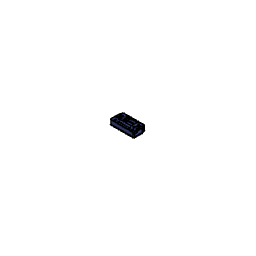
Remote (Autodesk Fusion 360 design; units mm, degrees)
Autodesk Fusion 360 part; units mm, degrees
(part 1 of 2)
sketch "Top" plane through (0, 0, 0) normal (0, 0, 1) x (1, 0, 0) in component "Case"
  line L0 (48, 28.17) -> (-50, 28.17) construction
  line L1 (-1, 28.17) -> (-1, -28.17) construction
  line L2 (-40, 26) -> (40, 26)
  circle A0 centre (45, -24.75) radius 3
  circle A1 centre (-47, -24.75) radius 1.3
  circle A2 centre (-47, -24.75) radius 3
  circle A3 centre (45, 24.75) radius 3
  line L3 (48, -28.17) -> (48, 28.17) construction
  circle A4 centre (-47, 24.75) radius 1.3
  line L4 (-50, -28.17) -> (48, -28.17) construction
  line L5 (40, 26) -> (40, -26)
  line L6 (40, -26) -> (-40, -26)
  circle A5 centre (45, -24.75) radius 1.3
  circle A6 centre (45, 24.75) radius 1.3
  line L7 (-40, -26) -> (-40, 26)
  line L8 (-50, 28.17) -> (-50, -28.17) construction
  circle A7 centre (-47, 24.75) radius 3
  line L9 (40, 0) -> (-40, 0) construction
  line L10 (-92, 15.5) -> (-92, -11.5) construction
  line L11 (-58, -11.5) -> (-92, 15.5) construction
  line L12 (-58, -11.5) -> (-58, 15.5) construction
  circle A8 centre (-75, 3) radius 11
  circle A9 centre (-62, -8) radius 2.5
  circle A10 centre (-88, -8) radius 2.5
  circle A11 centre (-88, 12) radius 2.5
  line L13 (-92, -11.5) -> (-58, -11.5) construction
  circle A12 centre (-88, 12) radius 1.25
  line L14 (-92, -11.5) -> (-58, 15.5) construction
  line L15 (-58, 2) -> (-92, 2) construction
  line L16 (-58, 15.5) -> (-92, 15.5) construction
  circle A13 centre (-62, 12) radius 1.25
  circle A14 centre (-88, -8) radius 1.25
  circle A15 centre (-62, -8) radius 1.25
  circle A16 centre (-62, 12) radius 2.5
  line L17 (-75, 15.5) -> (-75, -11.5) construction
  line L18 (1.75, 0) -> (22.5, 0)
  line L19 (0, 1.75) -> (0, 22.5)
  circle A17 centre (-45, -50) radius 3.625
  circle A18 centre (-45, -50) radius 9 construction
  line L20 (-75, 40) -> (-75, -70) construction
  circle A19 centre (-75, -50) radius 9 construction
  line L21 (-75, 10) -> (-75, -100) construction
  circle A20 centre (-75, -50) radius 3.625
  circle A21 centre (45, -50) radius 9 construction
  circle A22 centre (45, -50) radius 3.625
  circle A23 centre (75, -50) radius 9 construction
  circle A24 centre (75, -50) radius 3.625
  line L22 (-75, -50) -> (75, -50) construction
  circle A25 centre (-87, -23) radius 8
  circle A26 centre (-8, -50) radius 3.125
  circle A27 centre (87, -23) radius 8
  circle A28 centre (8, -50) radius 3.125
  line L23 (100, -65) -> (-100, -65)
  line L24 (-100, -65) -> (-100, 35)
  line L25 (-100, 35) -> (100, 35)
  line L26 (100, 35) -> (100, -65)
  line L27 (100, -65) -> (-100, 35) construction
  line L28 (-100, -65) -> (100, 35) construction
  circle A29 centre (62, -6) radius 2.5
  circle A30 centre (75, 5) radius 11
  line L29 (92, -9.5) -> (92, 17.5) construction
  circle A31 centre (88, 14) radius 1.25
  circle A32 centre (88, 14) radius 2.5
  line L30 (58, 17.5) -> (58, -9.5) construction
  circle A33 centre (88, -6) radius 2.5
  line L31 (58, -9.5) -> (92, -9.5) construction
  circle A34 centre (88, -6) radius 1.25
  line L32 (58, -9.5) -> (92, 17.5) construction
  circle A35 centre (62, 14) radius 2.5
  line L33 (92, 17.5) -> (58, 17.5) construction
  line L34 (92, 4) -> (58, 4) construction
  circle A36 centre (62, 14) radius 1.25
  line L35 (75, 17.5) -> (75, -9.5) construction
  circle A37 centre (62, -6) radius 1.25
  line L36 (92, -9.5) -> (58, 17.5) construction
  circle A38 centre (-63, -23) radius 8
  circle A39 centre (63, -23) radius 8
  circle A40 centre (-23, -50) radius 3.125
  circle A41 centre (23, -50) radius 3.125
  circle A42 centre (-55, 25) radius 3.125
  circle A43 centre (55, 25) radius 3.125
  line L37 (-43.5, -42.95) -> (-46.5, -42.95)
  line L38 (-46.5, -42.95) -> (-46.5, -41.45)
  line L39 (-46.5, -41.45) -> (-43.5, -41.45)
  line L40 (-43.5, -41.45) -> (-43.5, -42.95)
  line L41 (-43.5, -42.95) -> (-46.5, -41.45) construction
  line L42 (-46.5, -42.95) -> (-43.5, -41.45) construction
  line L43 (-36.45, -51.5) -> (-37.95, -51.5)
  line L44 (-37.95, -51.5) -> (-37.95, -48.5)
  line L45 (-37.95, -48.5) -> (-36.45, -48.5)
  line L46 (-36.45, -48.5) -> (-36.45, -51.5)
  line L47 (-36.45, -51.5) -> (-37.95, -48.5) construction
  line L48 (-37.95, -51.5) -> (-36.45, -48.5) construction
  line L49 (-43.5, -58.55) -> (-43.5, -57.05)
  line L50 (-46.5, -58.55) -> (-43.5, -58.55)
  line L51 (-46.5, -57.05) -> (-46.5, -58.55)
  line L52 (-43.5, -57.05) -> (-46.5, -57.05)
  line L53 (-73.75, -44.25) -> (-76.25, -44.25)
  line L54 (-76.25, -44.25) -> (-76.25, -42.75)
  line L55 (-76.25, -42.75) -> (-73.75, -42.75)
  line L56 (-73.75, -42.75) -> (-73.75, -44.25)
  line L57 (-73.75, -44.25) -> (-76.25, -42.75) construction
  line L58 (-76.25, -44.25) -> (-73.75, -42.75) construction
  line L59 (-45, -59) -> (-45, -41) construction
  line L60 (-52.05, -48.5) -> (-53.55, -48.5)
  line L61 (-52.05, -51.5) -> (-52.05, -48.5)
  line L62 (-53.55, -48.5) -> (-53.55, -51.5)
  line L63 (-53.55, -51.5) -> (-52.05, -51.5)
  line L64 (0, 1.75) -> (0, 22.5) construction
  line L65 (76.25, -42.75) -> (73.75, -42.75)
  line L66 (76.25, -44.25) -> (76.25, -42.75)
  line L67 (73.75, -44.25) -> (76.25, -44.25)
  line L68 (73.75, -42.75) -> (73.75, -44.25)
  line L69 (46.5, -41.45) -> (43.5, -41.45)
  line L70 (46.5, -42.95) -> (46.5, -41.45)
  line L71 (43.5, -42.95) -> (46.5, -42.95)
  line L72 (43.5, -41.45) -> (43.5, -42.95)
  line L73 (37.95, -51.5) -> (37.95, -48.5)
  line L74 (36.45, -48.5) -> (36.45, -51.5)
  line L75 (37.95, -48.5) -> (36.45, -48.5)
  line L76 (36.45, -51.5) -> (37.95, -51.5)
  line L77 (52.05, -51.5) -> (52.05, -48.5)
  line L78 (52.05, -48.5) -> (53.55, -48.5)
  line L79 (53.55, -48.5) -> (53.55, -51.5)
  line L80 (53.55, -51.5) -> (52.05, -51.5)
  line L81 (43.5, -57.05) -> (46.5, -57.05)
  line L82 (46.5, -57.05) -> (46.5, -58.55)
  line L83 (46.5, -58.55) -> (43.5, -58.55)
  line L84 (43.5, -58.55) -> (43.5, -57.05)
  line L85 (-87, -23) -> (-63, -23) construction
  line L86 (82, -43) -> (68, -43)
  line L87 (68, -43) -> (68, -57)
  line L88 (68, -57) -> (82, -57)
  line L89 (82, -57) -> (82, -43)
  line L90 (82, -43) -> (68, -57) construction
  line L91 (68, -43) -> (82, -57) construction
  line L92 (-68, -57) -> (-82, -57)
  line L93 (-68, -43) -> (-68, -57)
  line L94 (-82, -57) -> (-82, -43)
  line L95 (-82, -43) -> (-68, -43)
  point P0 (-75, 2)
  point P1 (-75, 2)
  point P2 (0, -15)
  point P3 (75, 4)
  point P4 (75, 4)
  point P5 (74.877, 10)
  point P6 (-45, -42.2)
  point P7 (-37.2, -50)
  point P8 (-75, -43.5)
  point P9 (75, -50)
  dimension "d1592" = 80
  dimension "d1593" = 52
  dimension "d1594" = 98
  dimension "d1595" = 56.34
  dimension "d1596" = 2.6
  dimension "d1597" = 3.42
  dimension "d1598" = 3
  dimension "d1607" = 6
  dimension "d1608" = 34
  dimension "d1609" = 27
  dimension "d1610" = 5
  dimension "d1611" = 2.5
  dimension "d1612" = 10
  dimension "d1613" = 13
  dimension "d1614" = 22
  dimension "d1615" = 1
  dimension "d1616" = 28.17
  dimension "d1617" = 50
  dimension "d1618" = 40
  dimension "d1619" = 35
  dimension "d1629" = 7.25
  dimension "d1630" = 18
  dimension "d1632" = 7.25
  dimension "d1633" = 18
  dimension "d1634" = 16
  dimension "d1635" = 6.25
  dimension "d1638" = 30
  dimension "d1641" = 200
  dimension "d1642" = 100
  dimension "d1650" = 32
  dimension "d1651" = 15
  dimension "d1652" = 35
  dimension "d1653" = 34
  dimension "d1654" = 27
  dimension "d1655" = 5
  dimension "d1656" = 2.5
  dimension "d1657" = 10
  dimension "d1658" = 13
  dimension "d1659" = 22
  dimension "d1660" = 1
  dimension "d1661" = 35
  dimension "d1817" = 12
  dimension "d1819" = 58
  dimension "d1820" = 25
  dimension "d1821" = 6.25
  dimension "d1822" = 22
  dimension "d1823" = 15
  dimension "d1824" = 6.25
  dimension "d1825" = 10
  dimension "d1826" = 45
  dimension "d1853" = 3
  dimension "d1854" = 1.5
  dimension "d1855" = 7.8
  dimension "d1856" = 1.5
  dimension "d1857" = 3
  dimension "d1858" = 7.8
  dimension "d1859" = 2.5
  dimension "d1860" = 1.5
  dimension "d1861" = 6.5
  dimension "d1864" = 14
  dimension "d1865" = 14
  constraint horizontal L2
  constraint vertical L5
  constraint horizontal L6
  constraint vertical L7
  constraint midpoint L9.start L5
  constraint midpoint L9.end L7
  constraint horizontal L0
  constraint perpendicular L0 L8
  constraint parallel L0 L4
  constraint parallel L3 L8
  constraint symmetric A5 A6 L9
  constraint concentric A0 A5
  constraint symmetric A0 A3 L9
  constraint midpoint L1.start L0
  constraint midpoint L1.end L4
  constraint symmetric L1 A1 A5
  constraint symmetric L1 A4 A6
  constraint symmetric L1 A0 A2
  constraint symmetric L1 A3 A7
  constraint perpendicular L12 L13
  constraint parallel L13 L16
  constraint parallel L10 L12
  constraint concentric A9 A15
  constraint symmetric A9 A10 L17
  constraint symmetric A14 A15 L17
  constraint symmetric A9 L15 A16
  constraint symmetric L15 A13 A15
  constraint symmetric A10 A11 L15
  constraint symmetric A12 L15 A14
  constraint coincident A8.centre L17
  constraint coincident P1 L11
  constraint coincident P1 L14
  constraint coincident P1 L17
  constraint coincident L17.end L13
  constraint coincident L17.start L16
  constraint coincident L15.end L10
  constraint coincident L15.start L12
  constraint coincident P1 L15
  constraint perpendicular L10 L15
  constraint collinear L9 L18
  constraint concentric A17 A18
  constraint vertical L20
  constraint concentric A19 A20
  constraint vertical L21
  constraint symmetric L19 A17 A22
  constraint symmetric L19 A18 A21
  constraint symmetric L19 A19 A23
  constraint symmetric L19 A20 A24
  constraint coincident A19.centre A20.centre
  constraint coincident P9 A23.centre
  constraint coincident L22 A26.centre
  constraint coincident A17.centre L22
  constraint coincident L21 A19.centre
  constraint symmetric L19 A25 A27
  constraint symmetric L19 A26 A28
  constraint horizontal L23
  constraint perpendicular L23 L24
  constraint parallel L23 L25
  constraint parallel L24 L26
  constraint coincident L27 P2
  constraint coincident L28 P2
  constraint coincident L19 P2
  constraint parallel L10 L17
  constraint parallel L13 L18
  constraint perpendicular L29 L31
  constraint parallel L31 L33
  constraint parallel L29 L30
  constraint concentric A33 A34
  constraint symmetric A29 A33 L35
  constraint symmetric A34 L35 A37
  constraint symmetric A32 A33 L34
  constraint symmetric A31 A34 L34
  constraint symmetric A29 A35 L34
  constraint symmetric L34 A36 A37
  constraint coincident A30.centre L35
  constraint coincident P4 L36
  constraint coincident P4 L32
  constraint coincident P4 L35
  constraint coincident L35.end L31
  constraint coincident L35.start L33
  constraint coincident L34.end L30
  constraint coincident L34.start L29
  constraint coincident P4 L34
  constraint perpendicular L30 L34
  constraint parallel L30 L35
  constraint collinear L20 L21
  constraint symmetric L20 A25 A38
  constraint symmetric L19 A38 A39
  constraint coincident L22 A40.centre
  constraint symmetric L19 A40 A41
  constraint symmetric L19 A42 A43
  constraint horizontal L37
  constraint perpendicular L37 L38
  constraint parallel L37 L39
  constraint parallel L38 L40
  constraint coincident L41 P6
  constraint coincident L42 P6
  constraint horizontal L43
  constraint perpendicular L43 L44
  constraint parallel L43 L45
  constraint parallel L44 L46
  constraint coincident L47 P7
  constraint coincident L48 P7
  constraint coincident L22 P7
  constraint symmetric L22 L37.start L49.end
  constraint symmetric L22 L37.end L51.start
  constraint symmetric L22 L38.end L50.start
  constraint symmetric L22 L39.end L49.start
  constraint horizontal L53
  constraint perpendicular L53 L54
  constraint parallel L53 L55
  constraint parallel L54 L56
  constraint coincident L57 P8
  constraint coincident L58 P8
  constraint coincident L20 P8
  constraint coincident L21 P8
  constraint coincident A18 L59.start
  constraint coincident A18 L59.end
  constraint perpendicular L39 L59
  constraint symmetric L43.start L59 L62.end
  constraint symmetric L43.end L59 L61.start
  constraint symmetric L44.end L59 L60.start
  constraint symmetric L45.end L59 L60.end
  constraint symmetric L37.start L64 L71.start
  constraint symmetric L37.end L64 L70.start
  constraint symmetric L38.end L64 L69.start
  constraint symmetric L39.end L64 L69.end
  constraint symmetric L43.start L64 L74.end
  constraint symmetric L43.end L64 L73.start
  constraint symmetric L44.end L64 L73.end
  constraint symmetric L45.end L64 L74.start
  constraint symmetric L49.start L64 L83.end
  constraint symmetric L49.end L64 L81.start
  constraint symmetric L50.start L64 L82.end
  constraint symmetric L51.start L64 L81.end
  constraint symmetric L53.start L64 L67.start
  constraint symmetric L53.end L64 L66.start
  constraint symmetric L54.end L64 L65.start
  constraint symmetric L55.end L64 L65.end
  constraint symmetric L60.start L64 L77.end
  constraint symmetric L60.end L64 L78.end
  constraint symmetric L61.start L64 L77.start
  constraint symmetric L62.end L64 L79.end
  constraint coincident A25.centre L85.start
  constraint coincident A38.centre L85.end
  constraint horizontal L86
  constraint perpendicular L86 L87
  constraint parallel L86 L88
  constraint parallel L87 L89
  constraint coincident L90 P9
  constraint coincident L91 P9
  constraint symmetric L19 L86.start L94.end
  constraint symmetric L19 L86.end L93.start
  constraint symmetric L19 L87.end L92.start
  constraint symmetric L19 L88.end L92.end
  measures "d1592" distance of L2.start L2.end
  measures "d1593" distance of L2.start L6.end
  measures "d1594" distance of L3.start L4.start
  measures "d1595" distance of L0.end L4.start
  measures "d1596" diameter of A5
  measures "d1597" distance of A0.centre L4
  measures "d1598" distance of A0.centre L3
  measures "d1607" diameter of A0
  measures "d1608" distance of L12.end L10.start
  measures "d1609" distance of L12.end L11.start
  measures "d1610" diameter of A9
  measures "d1611" diameter of A15
  measures "d1612" distance of A9.centre L15
  measures "d1613" distance of A9.centre L17
  measures "d1614" diameter of A8
  measures "d1615" distance of A8.centre L15
  measures "d1616" distance of L0 L9
  measures "d1617" distance of L8 L19
  measures "d1618" distance of L7 L19
  measures "d1619" distance of L7 A8.centre
  measures "d1629" diameter of A17
  measures "d1630" diameter of A18
  measures "d1632" diameter of A20
  measures "d1633" diameter of A19
  measures "d1634" diameter of A25
  measures "d1635" diameter of A26
  measures "d1638" distance of A17.centre A19.centre
  measures "d1641" distance of L24.end L25.end
  measures "d1642" distance of L23.end L24.end
  measures "d1650" distance of A8.centre L25
  measures "d1651" distance of L22 L23
  measures "d1652" distance of L9 L25
  measures "d1653" distance of L30.start L29.end
  measures "d1654" distance of L29.start L29.end
  measures "d1655" diameter of A33
  measures "d1656" diameter of A34
  measures "d1657" distance of A33.centre L34
  measures "d1658" distance of A33.centre L35
  measures "d1659" diameter of A30
  measures "d1660" distance of A30.centre L34
  measures "d1661" distance of L5 A30.centre
  measures "d1817" distance of L20 A25.centre
  measures "d1819" distance of A25.centre L25
  measures "d1820" distance of L20 L24
  measures "d1821" diameter of A40
  measures "d1822" distance of A17.centre A40.centre
  measures "d1823" distance of A26.centre A40.centre
  measures "d1824" diameter of A42
  measures "d1825" distance of L25 A42.centre
  measures "d1826" distance of L24 A42.centre
  measures "d1853" distance of L38.end L39.end
  measures "d1854" distance of L37.end L38.end
  measures "d1855" distance of A17.centre P6
  measures "d1856" distance of L44.end L45.end
  measures "d1857" distance of L43.end L44.end
  measures "d1858" distance of A17.centre P7
  measures "d1859" distance of L54.end L55.end
  measures "d1860" distance of L53.end L54.end
  measures "d1861" distance of A19.centre P8
  measures "d1864" distance of L87.end L88.end
  measures "d1865" distance of L86.end L87.end
extrude "Extrude1" add sketch "Top" against normal blind 38 contours L2 L5 L6 L7 | A0 | A1 | A2 | A3 | A4 | A5 | A6 | A7 | A8 | A9 | A10 | A11 | A12 | A13 | A14 | A15 | A16 | A17 | A20 | A22 | A24 | A25 | A26 | A27 | A28 | L23 L24 L25 L26 | A29 | A30 | A31 | A32 | A33 | A34 | A35 | A36 | A37 | A38 | A39 | A40 | A41 | A42 | A43 | L37 L38 L39 L40 | L43 L44 L45 L46 | L49 L50 L51 L52 | L53 L54 L56 L92 L93 L94 L95 | L53 L54 L56 L95 | L54 L55 L56 L95 | L60 L61 L62 L63 | L65 L66 L68 L86 | L66 L67 L68 L86 L87 L88 L89 | L66 L67 L68 L86 | L69 L70 L71 L72 | L73 L74 L75 L76 | L77 L78 L79 L80 | L81 L82 L83 L84 makes body 1 in component "Case"
sketch "Front" plane through (0, -65, 0) normal (0, -1, 0) x (1, 0, 0) in component "Case"
  line L0 (100, 0) -> (-100, 0)
  line L1 (-100, 0) -> (-100, -38)
  line L2 (-100, -38) -> (100, -38)
  line L3 (100, -38) -> (100, 0)
  circle A0 centre (97.5, -10) radius 2.5
  line L4 (100, 0) -> (100, -38) construction
  line L5 (100, 0) -> (0, 0) construction
  circle A1 centre (97.5, -10) radius 3.7
  line L6 (93.8001, -10.0324) -> (93.8001, 0)
  dimension "d1842" = 5
  dimension "d1843" = 2.5
  dimension "d1844" = 10
  dimension "d1845" = 7.4
  constraint coincident L0.start L3.end
  constraint coincident L2.end L3.start
  constraint coincident L5.end origin
  constraint concentric A0 A1
  constraint vertical L6
  constraint coincident A1 L6.start
  constraint coincident L5 L6.end
  measures "d1842" diameter of A0
  measures "d1843" distance of A0.centre L4
  measures "d1844" distance of A0.centre L5
  measures "d1845" diameter of A1
chamfer "Chamfer2" distance 10 distance2 30 1 edges at (100, 35, -19) measured on face at (-33.3333, 35, -12.6667) on bodies 1 in component "Case"
chamfer "Chamfer3" distance 30 distance2 10 1 edges at (-100, 35, -19) measured on face at (-100, -31.6667, -12.6667) on bodies 1 in component "Case"
fillet "Fillet4" radius 5 6 edges at (100, -65, -19) (-100, -65, -19) (90, 35, -19) (100, 5, -19) (-90, 35, -19) (-100, 5, -19) on bodies 1 in component "Case"
shell "Shell1" thickness 2.7 outward yes removed faces 1 at (31.6667, -18.8743, -38) on bodies 1 in component "Case"
extrude "Extrude2" cut sketch "Top" along normal blind 10 contours L2 L5 L6 L7 | A8 | A17 | A20 | A22 | A24 | A25 | A26 | A27 | A28 | A30 | A38 | A39 | A40 | A41 | A42 | A43 bodies 1 in component "Case"
extrude "Extrude4" add sketch "Top" against normal blind 4 contours A0 | A2 | A3 | A7 bodies 1 in component "Case"
extrude "Extrude5" add sketch "Top" against normal blind 17 contours A9 | A10 | A11 | A16 | A29 | A32 | A33 | A35 bodies 1 in component "Case"
extrude "Extrude15" cut sketch "Top" along normal blind 2.1 contours L37 L38 L39 L40 | L43 L44 L45 L46 | L49 L50 L51 L52 | L53 L54 L56 L95 | L54 L55 L56 L95 | L60 L61 L62 L63 | L65 L66 L68 L86 | L66 L67 L68 L86 | L69 L70 L71 L72 | L73 L74 L75 L76 | L77 L78 L79 L80 | L81 L82 L83 L84 bodies 1 in component "Case"
extrude "Extrude16" add sketch "Top" against normal blind 1.8 contours L53 L54 L56 L92 L93 L94 L95 | L66 L67 L68 L86 L87 L88 L89 bodies 1 in component "Case"
sketch "Left" plane through (-100, 0, 0) normal (1, 0, 0) x (0, 1, 0) in component "Case"
  line L0 (4.1886, 0) -> (-60, 0)
  line L1 (-60, -38) -> (4.1886, -38)
  line L2 (-60, 0) -> (4.1886, 0) construction
  line L3 (4.1886, 0) -> (4.1886, -38) construction
  line L4 (4.1886, -38) -> (-60, -38) construction
  line L5 (-60, -38) -> (-60, 0) construction
  line L6 (-37.9057, -38) -> (-17.9057, -38)
  line L7 (-17.9057, -38) -> (-17.9057, -32.6)
  line L8 (-17.9057, -32.6) -> (-37.9057, -32.6)
  line L9 (-37.9057, -32.6) -> (-37.9057, -38)
  line L10 (-60, 0) -> (-60, -38)
  line L11 (4.1886, -38) -> (4.1886, 0)
  point P0 (-27.9057, -38)
  point P1 (-27.9057, -38)
  dimension "d1712" = 20
  dimension "d1713" = 5.4
  constraint horizontal L2
  constraint vertical L3
  constraint horizontal L4
  constraint vertical L5
  constraint coincident L1.end L3.end
  constraint coincident L0.end L2.start
  constraint horizontal L6
  constraint vertical L7
  constraint horizontal L8
  constraint vertical L9
  constraint coincident L4 L6.start
  constraint midpoint L6 P1
  constraint midpoint L4 P1
  constraint coincident P1 P0
  measures "d1712" distance of L6.start L6.end
  measures "d1713" distance of L6.start L8.end
sketch "Back" plane through (0, 35, 0) normal (0, -1, 0) x (1, 0, 0) in component "Case"
  line L0 (86.3962, 0) -> (-86.3962, 0)
  line L1 (-86.3962, -38) -> (86.3962, -38)
  line L2 (-86.3962, 0) -> (86.3962, 0) construction
  line L3 (86.3962, 0) -> (86.3962, -38) construction
  line L4 (86.3962, -38) -> (-86.3962, -38) construction
  line L5 (-86.3962, -38) -> (-86.3962, 0) construction
  line L6 (2.8, -6.3) -> (2.8, -8.7)
  line L7 (5.5, -9.3) -> (5.5, -8.7)
  line L8 (5.5, -5.7) -> (5.5, -6.3)
  line L9 (4, -8.7) -> (4, -9.3)
  line L10 (4, -6.3) -> (4, -5.7)
  line L11 (2.5, -5.7) -> (2.5, -9.3)
  line L12 (19.5, -8.7) -> (19.5, -9.3)
  line L13 (27, -8.7) -> (28.2, -8.7)
  line L14 (11.5, -8.7) -> (11.5, -9.3)
  line L15 (18, -5.7) -> (18, -6.3)
  line L16 (28.2, -8.7) -> (28.2, -6.3)
  line L17 (25.5, -6.3) -> (19.5, -6.3)
  line L18 (11.5, -6.3) -> (11.5, -5.7)
  line L19 (15.5, -6.3) -> (15.5, -8.7) construction
  line L20 (13, -8.7) -> (18, -8.7)
  line L21 (19.5, -8.7) -> (25.5, -8.7)
  line L22 (25.5, -5.7) -> (25.5, -6.3)
  line L23 (25.5, -9.3) -> (25.5, -8.7)
  line L24 (28.2, -6.3) -> (27, -6.3)
  line L25 (18, -9.3) -> (18, -8.7)
  line L26 (19.5, -6.3) -> (19.5, -5.7)
  line L27 (4, -6.3) -> (2.8, -6.3)
  line L28 (2.8, -8.7) -> (4, -8.7)
  line L29 (5.5, -8.7) -> (11.5, -8.7)
  line L30 (27, -8.7) -> (27, -9.3)
  line L31 (27, -5.7) -> (25.5, -5.7)
  line L32 (28.2, -7.5) -> (2.8, -7.5) construction
  line L33 (28.5, -9.3) -> (28.5, -5.7)
  line L34 (18, -6.3) -> (13, -6.3)
  line L35 (13, -9.3) -> (13, -8.7)
  line L36 (13, -5.7) -> (13, -6.3)
  line L37 (19.5, -5.7) -> (18, -5.7)
  line L38 (27, -6.3) -> (27, -5.7)
  line L39 (28.5, -5.7) -> (2.5, -5.7)
  line L40 (11.5, -6.3) -> (5.5, -6.3)
  line L41 (2.5, -9.3) -> (28.5, -9.3)
  line L42 (-10, -38) -> (10, -38)
  line L43 (10, -38) -> (10, -32.6)
  line L44 (10, -32.6) -> (-10, -32.6)
  line L45 (-10, -32.6) -> (-10, -38)
  line L46 (50, -38) -> (70, -38)
  line L47 (70, -38) -> (70, -32.6)
  line L48 (70, -32.6) -> (50, -32.6)
  line L49 (50, -32.6) -> (50, -38)
  circle A0 centre (77.3962, -8.5) radius 6.25
  line L50 (0, 1.75) -> (0, 22.5)
  circle A1 centre (-77.3962, -8.5) radius 6.25
  line L51 (-70, -32.6) -> (-50, -32.6)
  line L52 (-70, -38) -> (-70, -32.6)
  line L53 (-50, -38) -> (-70, -38)
  line L54 (-50, -32.6) -> (-50, -38)
  line L55 (-86.3962, 0) -> (-86.3962, -38)
  line L56 (86.3962, -38) -> (86.3962, 0)
  line L57 (-49.3962, -8) -> (-40.3962, -8)
  line L58 (-40.3962, -8) -> (-40.3962, -22)
  line L59 (-40.3962, -22) -> (-49.3962, -22)
  line L60 (-49.3962, -22) -> (-49.3962, -8)
  line L61 (100, 0) -> (-100, 0)
  line L62 (1.75, 0) -> (22.5, 0)
  line L63 (39.3541, -17.5) -> (45.6541, -17.5) construction
  line L64 (42.5041, -20.65) -> (42.5041, -14.35) construction
  line L65 (41.7541, -14.4406) -> (41.7541, -15.1152)
  line L66 (39.4447, -16.75) -> (40.1193, -16.75)
  line L67 (39.4447, -18.25) -> (40.1193, -18.25)
  line L68 (41.7541, -20.5594) -> (41.7541, -19.8848)
  line L69 (43.2541, -14.4406) -> (43.2541, -15.1152)
  line L70 (45.5635, -16.75) -> (44.889, -16.75)
  line L71 (45.5635, -18.25) -> (44.889, -18.25)
  line L72 (43.2541, -20.5594) -> (43.2541, -19.8848)
  arc A2 (44.889, -16.75) -> (43.2541, -15.1152) centre (42.5041, -17.5) ccw
  arc A3 (43.2541, -19.8848) -> (44.889, -18.25) centre (42.5041, -17.5) ccw
  arc A4 (41.7541, -15.1152) -> (40.1193, -16.75) centre (42.5041, -17.5) ccw
  arc A5 (40.1193, -18.25) -> (41.7541, -19.8848) centre (42.5041, -17.5) ccw
  arc A6 (43.2541, -20.5594) -> (45.5635, -18.25) centre (42.5041, -17.5) ccw
  arc A7 (45.5635, -16.75) -> (43.2541, -14.4406) centre (42.5041, -17.5) ccw
  arc A8 (41.7541, -14.4406) -> (39.4447, -16.75) centre (42.5041, -17.5) ccw
  arc A9 (39.4447, -18.25) -> (41.7541, -20.5594) centre (42.5041, -17.5) ccw
  line L73 (-20, -7.25) -> (-20, -14.75)
  line L74 (-31, -14.75) -> (-31, -7.25)
  line L75 (-30.6, -7.85) -> (-30.6, -14.15)
  line L76 (-20.4, -14.15) -> (-20.4, -7.85)
  line L77 (-20.4, -7.85) -> (-30.6, -14.15) construction
  line L78 (-30.6, -7.85) -> (-20.4, -14.15) construction
  line L79 (-28.5, -7.25) -> (-28.5, -7.85)
  line L80 (-31, -11) -> (-20, -11) construction
  line L81 (-25.5, -14.75) -> (-25.5, -7.25) construction
  line L82 (-26.25, -7.85) -> (-26.25, -7.25)
  line L83 (-30, -7.25) -> (-30, -7.85)
  line L84 (-21, -7.25) -> (-21, -7.85)
  line L85 (-22.5, -7.25) -> (-22.5, -7.85)
  line L86 (-24.75, -7.85) -> (-24.75, -7.25)
  line L87 (-21, -14.75) -> (-21, -14.15)
  line L88 (-22.5, -14.75) -> (-22.5, -14.15)
  line L89 (-24.75, -14.15) -> (-24.75, -14.75)
  line L90 (-26.25, -14.15) -> (-26.25, -14.75)
  line L91 (-28.5, -14.75) -> (-28.5, -14.15)
  line L92 (-30, -14.75) -> (-30, -14.15)
  line L93 (-20.4, -7.85) -> (-21, -7.85)
  line L94 (-21, -7.25) -> (-20, -7.25)
  line L95 (-24.75, -7.25) -> (-22.5, -7.25)
  line L96 (-22.5, -7.85) -> (-24.75, -7.85)
  line L97 (-31, -7.25) -> (-30, -7.25)
  line L98 (-28.5, -7.25) -> (-26.25, -7.25)
  line L99 (-26.25, -7.85) -> (-28.5, -7.85)
  line L100 (-30, -7.85) -> (-30.6, -7.85)
  line L101 (-30.6, -14.15) -> (-30, -14.15)
  line L102 (-30, -14.75) -> (-31, -14.75)
  line L103 (-26.25, -14.75) -> (-28.5, -14.75)
  line L104 (-28.5, -14.15) -> (-26.25, -14.15)
  line L105 (-20, -14.75) -> (-21, -14.75)
  line L106 (-22.5, -14.75) -> (-24.75, -14.75)
  line L107 (-24.75, -14.15) -> (-22.5, -14.15)
  line L108 (-21, -14.15) -> (-20.4, -14.15)
  line L109 (100, 0) -> (100, -35) construction
  line L110 (-100, 0) -> (-100, -35) construction
  circle A10 centre (77.3962, -8.5) radius 8.25 construction
  circle A11 centre (77.3962, -26) radius 8.25
  circle A12 centre (77.3962, -26) radius 6.25
  circle A13 centre (-77.3962, -26) radius 8.25
  circle A14 centre (-77.3962, -26) radius 6.25
  circle A15 centre (-77.3962, -8.5) radius 8.25 construction
  line L111 (0, -840) -> (0, 760)
  point P0 (0, 1.5)
  point P1 (0, 1.5)
  point P2 (0, 1.5)
  point P3 (0, -38)
  point P4 (0, -38)
  point P5 (-25.5, -11)
  point P6 (-25.5, -11)
  point P7 (-25.5, -11)
  dimension "d1714" = 26
  dimension "d1715" = 3.6
  dimension "d1716" = 1.5
  dimension "d1717" = 0.6
  dimension "d1718" = 1.5
  dimension "d1719" = 2.5
  dimension "d1720" = 6
  dimension "d1721" = 2.5
  dimension "d1722" = 0.3
  dimension "d1723" = 0.3
  dimension "d1724" = 1.2
  dimension "d1725" = 0.6
  dimension "d1726" = 5.7
  dimension "d1727" = 20
  dimension "d1728" = 5.4
  dimension "d1729" = 20
  dimension "d1730" = 5.4
  dimension "d1732" = 12.5
  dimension "d1733" = 9
  dimension "d1734" = 8.5
  dimension "d1794" = 9
  dimension "d1795" = 14
  dimension "d1796" = 8
  dimension "d1797" = 37
  dimension "d1802" = 6.3
  dimension "d1803" = 5
  dimension "d1804" = 17.5
  dimension "d1805" = 0.75
  dimension "d1806" = 0.75
  dimension "d1807" = 11
  dimension "d1808" = 7.5
  dimension "d1810" = 11
  dimension "d1811" = 10.2
  dimension "d1812" = 6.3
  dimension "d1814" = 0.75
  dimension "d1815" = 1.5
  dimension "d1816" = 1
  dimension "d1818" = 74.5
  dimension "d1827" = 16.5
  dimension "d1828" = 12.5
  dimension "d1829" = 16.5
  dimension "d1830" = 17.5
  constraint horizontal L2
  constraint vertical L3
  constraint horizontal L4
  constraint vertical L5
  constraint coincident L1.end L3.end
  constraint coincident L0.end L2.start
  constraint coincident P2 P1
  constraint horizontal L39
  constraint vertical L11
  constraint horizontal L41
  constraint vertical L33
  constraint horizontal L31
  constraint vertical L22
  constraint vertical L38
  constraint coincident L31.start L39
  constraint midpoint L32.start L16
  constraint midpoint L32.end L6
  constraint horizontal L37
  constraint vertical L15
  constraint vertical L26
  constraint coincident L26.end L39
  constraint symmetric L10.end L31.start L19
  constraint symmetric L22.start L8.start L19
  constraint symmetric L8.end L17.start L19
  constraint symmetric L24.end L10.start L19
  constraint symmetric L18.end L26.end L19
  constraint symmetric L15.start L36.start L19
  constraint symmetric L15.end L34.end L19
  constraint symmetric L17.end L18.start L19
  constraint symmetric L31.start L30.end L32
  constraint symmetric L22.start L23.start L32
  constraint symmetric L17.start L21.end L32
  constraint symmetric L24.end L13.start L32
  constraint symmetric L26.end L12.end L32
  constraint symmetric L15.start L25.start L32
  constraint symmetric L15.end L20.end L32
  constraint symmetric L17.end L12.start L32
  constraint symmetric L10.start L9.start L32
  constraint symmetric L10.end L9.end L32
  constraint symmetric L8.start L7.start L32
  constraint symmetric L8.end L7.end L32
  constraint symmetric L18.start L14.start L32
  constraint symmetric L18.end L14.end L32
  constraint symmetric L36.start L35.start L32
  constraint symmetric L34.end L20.start L32
  constraint parallel L28 L41
  constraint parallel L16 L33
  constraint parallel L24 L39
  constraint parallel L6 L11
  constraint collinear L13 L28
  constraint coincident L19.end L28
  constraint collinear L21 L28
  constraint collinear L20 L28
  constraint collinear L28 L29
  constraint collinear L24 L27
  constraint coincident L19.start L24
  constraint collinear L24 L40
  constraint collinear L24 L34
  constraint collinear L17 L24
  constraint horizontal L42
  constraint vertical L43
  constraint horizontal L44
  constraint vertical L45
  constraint coincident L4 L42.start
  constraint midpoint L42 P4
  constraint midpoint L4 P4
  constraint coincident P4 P3
  constraint horizontal L46
  constraint vertical L47
  constraint horizontal L48
  constraint vertical L49
  constraint coincident L4 L46.start
  constraint symmetric L46.start L50 L53.start
  constraint symmetric L46.end L50 L52.start
  constraint symmetric L47.end L50 L51.start
  constraint symmetric L48.end L50 L51.end
  constraint symmetric A0 L50 A1
  constraint horizontal L57
  constraint vertical L58
  constraint horizontal L59
  constraint vertical L60
  constraint concentric A4 A8
  constraint coincident L63.start A8
  constraint coincident L63.end A8
  constraint parallel L17 L63
  constraint perpendicular L63 L64
  constraint parallel L64 L65
  constraint horizontal L66
  constraint symmetric L63 L65.start L68.start
  constraint symmetric L63 L65.end L68.end
  constraint symmetric L63 L66.start L67.start
  constraint symmetric L63 L66.end L67.end
  constraint symmetric L64 L65.start L69.start
  constraint symmetric L64 L65.end L69.end
  constraint symmetric L64 L66.start L70.start
  constraint symmetric L64 L66.end L70.end
  constraint symmetric L64 L67.start L71.start
  constraint symmetric L64 L67.end L71.end
  constraint symmetric L64 L68.start L72.start
  constraint symmetric L64 L68.end L72.end
  constraint concentric A2 A4
  constraint concentric A3 A4
  constraint concentric A6 A8
  constraint concentric A4 A5
  constraint concentric A6 A7
  constraint concentric A8 A9
  constraint horizontal L97
  constraint vertical L73
  constraint horizontal L105
  constraint vertical L74
  constraint horizontal L93
  constraint perpendicular L75 L93
  constraint parallel L93 L101
  constraint parallel L75 L76
  constraint coincident L77 P7
  constraint coincident L78 P7
  constraint coincident P7 P6
  constraint coincident L79.start L97
  constraint coincident L79.end L93
  constraint perpendicular L79 L93
  constraint midpoint L74 L80.start
  constraint midpoint L73 L80.end
  constraint coincident L82.start L93
  constraint perpendicular L82 L97
  constraint midpoint L80 P7
  constraint coincident L83.end L93
  constraint perpendicular L83 L93
  constraint symmetric L79.start L81 L85.start
  constraint symmetric L79.end L81 L85.end
  constraint symmetric L81 L82.start L86.start
  constraint symmetric L81 L82.end L86.end
  constraint symmetric L81 L83.start L84.start
  constraint symmetric L81 L83.end L84.end
  constraint symmetric L79.start L80 L91.start
  constraint symmetric L79.end L80 L91.end
  constraint symmetric L80 L82.start L90.start
  constraint symmetric L80 L82.end L90.end
  constraint symmetric L80 L83.start L92.start
  constraint symmetric L80 L83.end L92.end
  constraint symmetric L80 L84.start L87.start
  constraint symmetric L80 L84.end L87.end
  constraint symmetric L80 L85.start L88.start
  constraint symmetric L80 L85.end L88.end
  constraint symmetric L80 L86.start L89.start
  constraint symmetric L80 L86.end L89.end
  constraint collinear L93 L96
  constraint collinear L94 L97
  constraint collinear L95 L97
  constraint collinear L96 L99
  constraint collinear L97 L98
  constraint collinear L99 L100
  constraint collinear L101 L104
  constraint collinear L102 L105
  constraint coincident L81.start L105
  constraint collinear L103 L105
  constraint collinear L104 L107
  constraint collinear L105 L106
  constraint collinear L107 L108
  constraint coincident L61.start L109.start
  constraint perpendicular L61 L109
  constraint coincident L61.end L110.start
  constraint perpendicular L61 L110
  constraint concentric A0 A10
  constraint concentric A11 A12
  constraint symmetric L50 A10 A15
  constraint symmetric L50 A11 A13
  constraint symmetric L50 A12 A14
  measures "d1714" distance of L33.end L11.start
  measures "d1715" distance of L33.start L33.end
  measures "d1716" distance of L22.start L31.start
  measures "d1717" distance of L17.start L22.start
  measures "d1718" distance of L26.end L15.start
  measures "d1719" distance of L15 L19
  measures "d1720" distance of L22 L26
  measures "d1721" distance of P2 L11
  measures "d1722" distance of L16 L33
  measures "d1723" distance of L6 L11
  measures "d1724" distance of L6.start L10.start
  measures "d1725" distance of L21 L41
  measures "d1726" distance of L2 L39
  measures "d1727" distance of L42.start L42.end
  measures "d1728" distance of L42.start L44.end
  measures "d1729" distance of L46.start L46.end
  measures "d1730" distance of L46.start L48.end
  measures "d1732" diameter of A0
  measures "d1733" distance of L3 A0.centre
  measures "d1734" distance of L2 A0.centre
  measures "d1794" distance of L57.start L57.end
  measures "d1795" distance of L57.start L59.end
  measures "d1796" distance of L57 L61
  measures "d1797" distance of L5 L60
  measures "d1802" diameter of A8
  measures "d1803" diameter of A4
  measures "d1804" distance of A2.centre L62
  measures "d1805" distance of L64 L65
  measures "d1806" distance of L63 L66
  measures "d1807" distance of L74.end L73.start
  measures "d1808" distance of L74.end L74.start
  measures "d1810" distance of L2 P7
  measures "d1811" distance of L75.end L76.start
  measures "d1812" distance of L75.start L75.end
  measures "d1814" distance of L81 L82
  measures "d1815" distance of L79 L83
  measures "d1816" distance of L74 L83
  measures "d1818" distance of P7 L110
  measures "d1827" diameter of A10
  measures "d1828" diameter of A12
  measures "d1829" diameter of A11
  measures "d1830" distance of A0.centre A11.centre
extrude "Extrude6" cut sketch "Back" against normal blind 3 contours L6 L9 L10 L11 L27 L28 L39 L41 | L8 L18 L39 L40 | L7 L14 L29 L41 | L15 L34 L36 L39 | L20 L25 L35 L41 | L17 L22 L26 L39 | L12 L21 L23 L41 | L13 L16 L24 L30 L33 L38 L39 L41 | A0 | A1 | L57 L58 L59 L60 | L65 L66 A4 A8 | L67 L68 A5 A9 | L69 L70 A2 A7 | L71 L72 A3 A6 | L73 L76 L84 L87 L93 L94 L105 L108 | L74 L75 L83 L92 L97 L100 L101 L102 | L79 L82 L98 L99 | L85 L86 L95 L96 | L88 L89 L106 L107 | L90 L91 L103 L104 | A12 | A14 bodies 1 in component "Case"
extrude "Extrude7" add sketch "Back" along normal blind 4 draft -45 contours L1 L46 L47 L48 L49 | L1 L42 L44 L45 L111 | L1 L42 L43 L44 L111 | L1 L51 L52 L53 L54 bodies 1 in component "Case"
extrude "Extrude8" add sketch "Left" along normal blind 5 draft -45 contours L1 L6 L7 L8 L9 bodies 1 in component "Case"
mirror "Mirror1" about plane through (0, 0, 0) normal (1, 0, 0) of "Extrude8" in component "Case"
ref_plane "WorkPlane1" through (0, -15, -19) normal (0, 1, 0) x (1, 0, 0) in component "Case"
mirror "Mirror2" about plane through (0, -15, -19) normal (0, 1, 0) of "Extrude7" in component "Case"
sketch "Sketch1" plane through (0, 0, -38) normal (0, 0, -1) x (1, 0, 0) in component "Cover (2)"
  line L0 (-100, -4.1886) -> (-100, 17.9057)
  line L1 (-100, 17.9057) -> (-100, 37.9057)
  line L2 (-100, 37.9057) -> (-100, 60)
  line L3 (-95, 65) -> (-70, 65)
  line L4 (-70, 65) -> (-50, 65)
  line L5 (-50, 65) -> (-10, 65)
  line L6 (-10, 65) -> (10, 65)
  line L7 (10, 65) -> (50, 65)
  line L8 (50, 65) -> (70, 65)
  line L9 (70, 65) -> (95, 65)
  line L10 (100, 60) -> (100, 37.9057)
  line L11 (100, 37.9057) -> (100, 17.9057)
  line L12 (100, 17.9057) -> (100, -4.1886)
  line L13 (86.3962, -35) -> (70, -35)
  line L14 (70, -35) -> (50, -35)
  line L15 (50, -35) -> (10, -35)
  line L16 (10, -35) -> (-10, -35)
  line L17 (-10, -35) -> (-50, -35)
  line L18 (-50, -35) -> (-70, -35)
  line L19 (-70, -35) -> (-86.3962, -35)
  line L20 (95, 67.7) -> (-95, 67.7)
  line L21 (-102.7, 60) -> (-102.7, -4.1886)
  line L22 (-86.3962, -37.7) -> (86.3962, -37.7)
  line L23 (102.7, -4.1886) -> (102.7, 60)
  arc A0 (-95, 65) -> (-100, 60) centre (-95, 60) ccw
  arc A1 (100, 60) -> (95, 65) centre (95, 60) ccw
  arc A2 (102.7, 60) -> (95, 67.7) centre (95, 60) ccw
  arc A3 (-95, 67.7) -> (-102.7, 60) centre (-95, 60) ccw
  arc A4 (99.7434, -5.7698) -> (100, -4.1886) centre (95, -4.1886) ccw
  line L24 (99.7434, -5.7698) -> (91.1396, -31.5811)
  arc A5 (86.3962, -35) -> (91.1396, -31.5811) centre (86.3962, -30) ccw
  arc A6 (-91.1396, -31.5811) -> (-86.3962, -35) centre (-86.3962, -30) ccw
  line L25 (-91.1396, -31.5811) -> (-99.7434, -5.7698)
  arc A7 (-100, -4.1886) -> (-99.7434, -5.7698) centre (-95, -4.1886) ccw
  arc A8 (-102.7, -4.1886) -> (-102.3049, -6.6236) centre (-95, -4.1886) ccw
  line L26 (-102.3049, -6.6236) -> (-93.7011, -32.435)
  arc A9 (-93.7011, -32.435) -> (-86.3962, -37.7) centre (-86.3962, -30) ccw
  arc A10 (86.3962, -37.7) -> (93.7011, -32.435) centre (86.3962, -30) ccw
  line L27 (93.7011, -32.435) -> (102.3049, -6.6236)
  arc A11 (102.3049, -6.6236) -> (102.7, -4.1886) centre (95, -4.1886) ccw
extrude "Extrude1'" add sketch "Sketch1" along normal blind 2.7 separate body contours L0 L1 L2 L3 L4 L5 L6 L7 L8 L9 L10 L11 L12 L13 L14 L15 L16 L17 L18 L19 A0 A1 A4 L24 A5 A6 L25 A7 | L20 L21 L22 L23 A2 A3 A8 L26 A9 A10 L27 A11 makes body 2 in component "Cover (2)"
sketch "Sketch2" plane through (0, 0, -38) normal (0, 0, 1) x (-1, 0, 0) in component "Cover (2)"
  line L0 (-102.7, 60) -> (-102.7, -4.1886)
  line L1 (-86.3962, -37.7) -> (86.3962, -37.7)
  line L2 (102.7, -4.1886) -> (102.7, 60)
  line L3 (95, 67.7) -> (-95, 67.7)
  arc A0 (102.7, 60) -> (95, 67.7) centre (95, 60) ccw
  arc A1 (-95, 67.7) -> (-102.7, 60) centre (-95, 60) ccw
  arc A2 (-102.7, -4.1886) -> (-102.3049, -6.6236) centre (-95, -4.1886) ccw
  line L4 (-102.3049, -6.6236) -> (-93.7011, -32.435)
  arc A3 (-93.7011, -32.435) -> (-86.3962, -37.7) centre (-86.3962, -30) ccw
  arc A4 (86.3962, -37.7) -> (93.7011, -32.435) centre (86.3962, -30) ccw
  line L5 (93.7011, -32.435) -> (102.3049, -6.6236)
  arc A5 (102.3049, -6.6236) -> (102.7, -4.1886) centre (95, -4.1886) ccw
  line L6 (-99.5537, -5.7065) -> (-90.9499, -31.5179)
  arc A6 (-90.9499, -31.5179) -> (-86.3962, -34.8) centre (-86.3962, -30) ccw
  line L7 (-86.3962, -34.8) -> (86.3962, -34.8)
  arc A7 (86.3962, -34.8) -> (90.9499, -31.5179) centre (86.3962, -30) ccw
  line L8 (90.9499, -31.5179) -> (99.5537, -5.7065)
  arc A8 (99.5537, -5.7065) -> (99.8, -4.1886) centre (95, -4.1886) ccw
  line L9 (99.8, -4.1886) -> (99.8, 60)
  arc A9 (99.8, 60) -> (95, 64.8) centre (95, 60) ccw
  line L10 (95, 64.8) -> (-95, 64.8)
  arc A10 (-95, 64.8) -> (-99.8, 60) centre (-95, 60) ccw
  line L11 (-99.8, 60) -> (-99.8, -4.1886)
  arc A11 (-99.8, -4.1886) -> (-99.5537, -5.7065) centre (-95, -4.1886) ccw
  line L12 (100, -37.7388) -> (-100, -37.7388) construction
  line L13 (-100, -37.7388) -> (-100, 61.9) construction
  line L14 (-100, 61.9) -> (100, 61.9) construction
  line L15 (100, 61.9) -> (100, -37.7388) construction
  circle A12 centre (60, -22.7388) radius 1.25
  circle A13 centre (60, -22.7388) radius 3
  line L16 (0, -1.75) -> (0, -22.5)
  line L17 (60, -37.7388) -> (60, 64.8) construction
  circle A14 centre (60, -2.7388) radius 1.25
  circle A15 centre (60, -2.7388) radius 3
  circle A16 centre (-60, -22.7388) radius 3
  circle A17 centre (-60, -22.7388) radius 1.25
  circle A18 centre (-60, -2.7388) radius 3
  circle A19 centre (-60, -2.7388) radius 1.25
  line L18 (80, 31.9) -> (-80, 31.9)
  line L19 (-80, 31.9) -> (-80, 61.9)
  line L20 (-80, 61.9) -> (80, 61.9)
  line L21 (80, 61.9) -> (80, 31.9)
  point P0 (0, 61.9)
  point P1 (0, 61.9)
  dimension "d1874" = 2.5
  dimension "d1875" = 6
  dimension "d1876" = 60
  dimension "d1877" = 15
  dimension "d1878" = 2.5
  dimension "d1879" = 6
  dimension "d1880" = 20
  dimension "d1909" = 160
  dimension "d1910" = 30
  dimension "d1913" = 2.9
  constraint horizontal L12
  constraint vertical L13
  constraint horizontal L14
  constraint vertical L15
  constraint concentric A12 A13
  constraint coincident L12 L17.start
  constraint coincident L10 L17.end
  constraint perpendicular L10 L17
  constraint coincident A12.centre L17
  constraint coincident L17 A14.centre
  constraint concentric A14 A15
  constraint symmetric A12 L16 A17
  constraint symmetric A13 L16 A16
  constraint symmetric L16 A14 A19
  constraint symmetric L16 A15 A18
  constraint horizontal L18
  constraint vertical L19
  constraint horizontal L20
  constraint vertical L21
  constraint midpoint L20 P1
  constraint midpoint L14 P1
  constraint coincident P1 P0
  constraint coincident L16 P1
  measures "d1874" diameter of A12
  measures "d1875" diameter of A13
  measures "d1876" distance of A12.centre L16
  measures "d1877" distance of L12 A12.centre
  measures "d1878" diameter of A14
  measures "d1879" diameter of A15
  measures "d1880" distance of A12.centre A14.centre
  measures "d1909" distance of L18.start L18.end
  measures "d1910" distance of L18.start L20.end
  measures "d1913" distance of L10 P1
extrude "Extrude2'" add sketch "Sketch2" along normal blind 5.4 contours L6 A6 L7 A7 L8 A8 L9 A9 L10 A10 L11 A11 | A12 | A13 | A14 | A15 | A16 | A17 | A18 | A19 | L18 L19 L20 L21 bodies 2 in component "Cover (2)"
extrude "Extrude3" cut sketch "Left" along normal blind 5 draft -45 from surface at 0.2 contours L1 L6 L7 L8 L9 bodies 2 in component "Cover (2)"
extrude "Extrude4'" cut sketch "Back" along normal blind 5 draft -45 from surface at 0.2 contours L1 L46 L47 L48 L49 | L1 L42 L44 L45 L111 | L1 L42 L43 L44 L111 | L1 L51 L52 L53 L54 bodies 2 in component "Cover (2)"
mirror "Mirror1'" about plane through (0, -15, -19) normal (0, 1, 0) of "Extrude4'" in component "Cover (2)"
mirror "Mirror2'" about plane through (0, 0, 0) normal (1, 0, 0) of "Extrude3" in component "Cover (2)"
shell "Shell2" thickness 2.7 removed faces 1 at (66.6, -15.9686, -32.6) on bodies 2 in component "Cover (2)"
chamfer "Chamfer1" distance 0.6 angle 45 8 edges at (-60, 34.8, -32.6) (-99.8, -27.9057, -32.6) (0, 34.8, -32.6) (60, 34.8, -32.6) (99.8, -27.9057, -32.6) (60, -64.8, -32.6) (0, -64.8, -32.6) (-60, -64.8, -32.6) on bodies 2 in component "Cover (2)"
chamfer "Chamfer1'" distance 1.8 angle 45 4 edges at (-40, 0, 2.7) (0, -26, 2.7) (40, 0, 2.7) (0, 26, 2.7) on bodies 1 in component "Case"
fillet "Fillet5" radius 2 12 edges at (102.7, -27.9057, 2.7) (100.4447, -65.4447, 2.7) (0, -67.7, 2.7) (-100.4447, -65.4447, 2.7) (-102.7, -27.9057, 2.7) (-102.6006, 5.422, 2.7) (-98.003, 19.5293, 2.7) (-90.8985, 36.2466, 2.7) (0, 37.7, 2.7) (90.8985, 36.2466, 2.7) (98.003, 19.5293, 2.7) (102.6006, 5.422, 2.7) on bodies 1 in component "Case"
fillet "Fillet2" radius 1.8 1 faces at (-28.7987, -32.5667, -40.7) on bodies 2 in component "Cover (2)"
sketch "Sketch5" plane through (0, 0, 0) normal (0, 0, 1) x (1, 0, 0) in component "Case"
sphere "SpherePrimitive1" add diameter 29 placed x (1, 0, 0) y (0, 1, 0) z (0, 0, 1) at (75, 5, 0) separate body makes body 3 in component "Case"
sphere "SpherePrimitive2" add diameter 29 placed x (1, 0, 0) y (0, 1, 0) z (0, 0, 1) at (-75, 5, 0) separate body makes body 4 in component "Case"
move_body "MoveFace1" bodies 3 4 to x (1, 0, 0) y (0, 1, 0) z (0, 0, 1) at (0, 0, -6) on bodies 3 4 in component "Case"
extrude "Extrude9" cut sketch "Top" along normal blind 10 contours A8 | L23 L24 L25 L26 | A30 | A38 | A39 | A40 | A41 | A42 | A43 | L37 L38 L39 L40 | L43 L44 L45 L46 | L49 L50 L51 L52 | L53 L54 L56 L92 L93 L94 L95 | L53 L54 L56 L95 | L54 L55 L56 L95 | L60 L61 L62 L63 | L65 L66 L68 L86 | L66 L67 L68 L86 L87 L88 L89 | L66 L67 L68 L86 | L69 L70 L71 L72 | L73 L74 L75 L76 | L77 L78 L79 L80 | L81 L82 L83 L84 bodies 3 4 in component "Case"
combine "Combine1" operation cut target body 1 tool bodies 3 4 in component "Case"
chamfer "Chamfer4" distance 1.8 distance2 2.4 2 edges at (64.7444, 8.9778, 2.7) (-78.9778, -7.2556, 2.7) measured on face at (-2.5888, -34.1612, 2.7) measured on face at (-2.5888, -34.1612, 2.7) on bodies 1 in component "Case"
extrude "Extrude5'" cut sketch "Back" along normal blind 5 contours A11 | A12 | A13 | A14 bodies 2 in component "Cover (2)"
extrude "Extrude6'" cut sketch "Back" against normal blind 5 contours A11 | A12 | A13 | A14 bodies 2 in component "Cover (2)"
sketch "TopTop" plane through (0, 0, 2.7) normal (0, 0, 1) x (-1, 0, 0) in component "Case"
  circle A0 centre (-75, -5) radius 12.8
  line L0 (41.8, 27.8) -> (41.8, -27.8)
  line L1 (41.8, -27.8) -> (-41.8, -27.8)
  line L2 (-41.8, -27.8) -> (-41.8, 27.8)
  line L3 (-41.8, 27.8) -> (41.8, 27.8)
  circle A1 centre (-55, -25) radius 3.125
  circle A2 centre (87, 23) radius 8
  circle A3 centre (-8, 50) radius 3.125
  circle A4 centre (-45, 50) radius 3.625
  circle A5 centre (75, 50) radius 3.625
  circle A6 centre (55, -25) radius 3.125
  circle A7 centre (-23, 50) radius 3.125
  circle A8 centre (63, 23) radius 8
  circle A9 centre (8, 50) radius 3.125
  circle A10 centre (-87, 23) radius 8
  circle A11 centre (-75, 50) radius 3.625
  circle A12 centre (45, 50) radius 3.625
  circle A13 centre (-63, 23) radius 8
  circle A14 centre (23, 50) radius 3.125
  line L4 (-100.7, 60) -> (-100.7, -4.1886)
  arc A15 (-100.7, -4.1886) -> (-100.4075, -5.9911) centre (-95, -4.1886) ccw
  line L5 (-100.4075, -5.9911) -> (-91.8037, -31.8025)
  arc A16 (-91.8037, -31.8025) -> (-86.3962, -35.7) centre (-86.3962, -30) ccw
  line L6 (-86.3962, -35.7) -> (86.3962, -35.7)
  arc A17 (86.3962, -35.7) -> (91.8037, -31.8025) centre (86.3962, -30) ccw
  line L7 (91.8037, -31.8025) -> (100.4075, -5.9911)
  arc A18 (100.4075, -5.9911) -> (100.7, -4.1886) centre (95, -4.1886) ccw
  line L8 (100.7, -4.1886) -> (100.7, 60)
  arc A19 (100.7, 60) -> (95, 65.7) centre (95, 60) ccw
  line L9 (95, 65.7) -> (-95, 65.7)
  arc A20 (-95, 65.7) -> (-100.7, 60) centre (-95, 60) ccw
  circle A21 centre (75, -3) radius 12.8
  circle A22 centre (-90, -24) radius 2.5
  circle A23 centre (-90, -24) radius 3.7
  dimension "d1835" = 5
  dimension "d1836" = 7.4
  constraint concentric A22 A23
  measures "d1835" diameter of A22
  measures "d1836" diameter of A23
extrude "Extrude10" add sketch "TopTop" against normal blind 30 contours A22 | A23 bodies 1 in component "Case"
extrude "Extrude11" cut sketch "TopTop" against normal blind 35 contours A22 bodies 1 in component "Case"
chamfer "Chamfer5" distance 2.7 angle 45 1 edges at (92.3308, 23.096, 2.7) on bodies 1 in component "Case"
extrude "Extrude12" add sketch "Front" against normal blind 32 contours A0 | L3 A1 | L0 L3 A1 L6 | L3 A1 bodies 1 in component "Case"
extrude "Extrude13" cut sketch "Front" along normal blind 10 contours A0 bodies 1 in component "Case"
extrude "Extrude14" cut sketch "Front" against normal blind 35 contours A0 bodies 1 in component "Case"
chamfer "Chamfer6" distance 2.7 angle 45 1 edges at (100, -65.8558, -10) on bodies 1 in component "Case"
extrude "Extrude7'" add sketch "Sketch2" along normal blind 6 contours A12 | A13 | A14 | A15 | A16 | A17 | A18 | A19 bodies 2 in component "Cover (2)"
extrude "Extrude8'" cut sketch "Sketch2" against normal blind 7.7 contours A12 | A14 | A17 | A19 bodies 2 in component "Cover (2)"